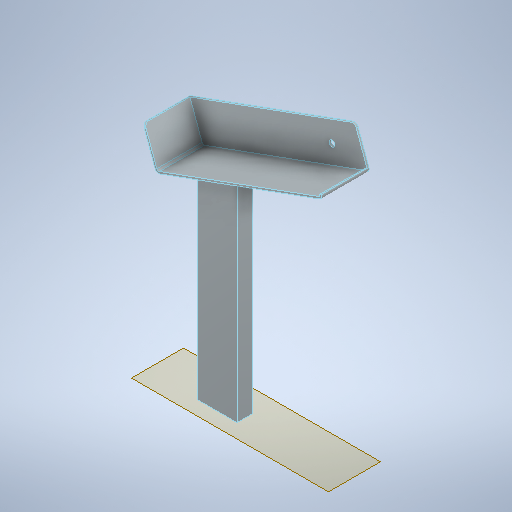
# Autodesk Inventor part: shooter base
Saved by Autodesk Inventor 2025.4 (Build 294407000, 407)
## iProperties
Created: 2026-03-09
Part Number: shooter base
Material: Stainless Steel
Document SubType Name: Modeling
Designer: youse
Density: 8 g/cm^3
Appearance: Turquoise
Author: youse
Finish1_Area: 14669.072 mm^2
Finish1_Appearance: Aluminum - Dark
Finish2_Area: 14669.072 mm^2
Finish2_Appearance: Zinc
Finish2_Process: Zn8/An
Finish2_Description: Zinc thickness 8μm, Transparent passivation
Finish2_ShortDescription: Zn8/An
Finish2_Thickness: 0.008 mm
## iProperties of the stored document shooter base_3DPrint.ipt
Created: 2026-03-12
Part Number: shooter base_3DPrint
Material: Generic
Document SubType Name: Modeling
Designer: youse
Density: 1 g/cm^3
Appearance: Default
Author: youse
Autodesk Inventor part; units mm, degrees
ref_plane "YZ Plane" through (0, 0, 0) normal (1, 0, 0) x (0, 1, 0)
ref_plane "XY Plane" through (0, 0, 0) normal (0, 0, 1) x (1, 0, 0)
sketch "Sketch1" plane through (0, 0, 0) normal (0, 0, 1) x (1, 0, 0)
  line L0 (1.879385, 0.68404) -> (82.692951, 30.097773)
  line L1 (0, 0) -> (86, 0) construction
  line L2 (83.888296, 32.661198) -> (77.731933, 49.575665)
  line L3 (77.731933, 49.575665) -> (-6.840403, 18.793852)
  line L4 (-6.840403, 18.793852) -> (-0.68404, 1.879385)
  arc A0 (-0.68404, 1.879385) -> (1.879385, 0.68404) centre (1.195345, 2.563426) ccw
  arc A1 (82.692951, 30.097773) -> (83.888296, 32.661198) centre (82.00891, 31.977158) ccw
  point P0 (84.572336, 30.781813)
  dimension "d0" = 90
  dimension "d1" = 20
  dimension "d2" = 20
  dimension "d9" = 2
  constraints: 10 end point, 4 point on circle, 4 point on line, 4 tangent, 3 perpendicular, 2 centre point, 1 equal length, 1 equal radius, 1 horizontal
  measures "d0" distance of L1.start point (84.572, 30.782)
  measures "d1" angle of L1 L0
  measures "d2" distance of point (84.572, 30.782) L2.end
  measures "d9" radius of A0
extrude "Extrusion1" add sketch "Sketch1" along normal blind 10 and the other way blind 13.991
shell "Shell1" thickness 1 removed faces 3 at (49.541154, 39.315061, -5.994) at (81.836175, 38.299354, 2.003) at (24.256972, 23.017853, 10)
fillet "Fillet1" radius 2 2 edges at (-6.3706, 18.9649, 10) (77.7319, 49.5757, -13.491)
sketch "Sketch2" plane through (1.537365, 1.623733, -12.991) normal (0, 0, 1) x (0.9396926, 0.3420201, 0)
  point P0 (-2, -1)
sketch "Sketch3" plane through (1.537365, 1.623733, -12.991) normal (0, 0, 1) x (0.9396926, 0.3420201, 0)
  circle A0 centre (72, 9) radius 1.5
  line L0 (88, 17) -> (88, 1) projected
  line L1 (86, 0) -> (0, 0) projected
  point P0 (-2, -1)
  dimension "d10" = 3
  dimension "d11" = 16
  dimension "d12" = 9
  constraints: 1 centre point
  measures "d10" diameter of A0
  measures "d11" distance from line of L0 A0.centre
  measures "d12" distance from line of L1 A0.centre
extrude "Extrusion2" cut sketch "Sketch3" against normal through all
ref_plane "Work Plane1" through (0, -95, 0) normal (0, 1, 0) x (-1, 0, 0)
sketch "Sketch4" plane through (0, -95, 0) normal (0, 1, 0) x (-1, 0, 0)
  line L0 (-15, -4) -> (-35, -4)
  line L1 (-35, -4) -> (-35, 4)
  line L2 (-35, 4) -> (-15, 4)
  line L3 (-15, 4) -> (-15, -4)
  point P0 (0, 0)
  point P1 (-25, 4)
  point P2 (-25, -4)
  dimension "d16" = 20
  dimension "d17" = 8
  dimension "d18" = 25
  dimension "d19" = 4
  constraints: 8 end point, 2 midpoint, 2 parallel, 1 horizontal, 1 perpendicular
  measures "d16" distance of L1.end L2.end
  measures "d17" distance of L0.end L1.end
  measures "d18" horizontal distance of point (0, 0) point (-25, 4)
  measures "d19" vertical distance of point (-25, -4) point (0, 0)
extrude "Extrusion3" add sketch "Sketch4" along normal up to surface surface through (1.879385, 0.68404, 0) normal (0.3420201, -0.9396926, 0)
body "Solid1"
